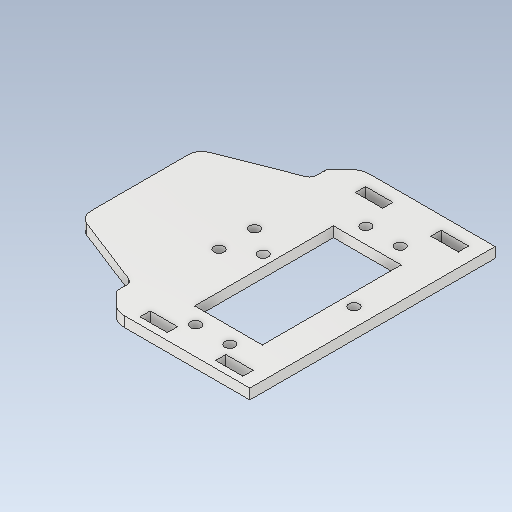
# Autodesk Inventor part: Dock bot2
Saved by Autodesk Inventor 2020.3 (Build 243373000, 373)
## iProperties
Created: 2017-03-28
Part Number: Dock bot2
Material: Acrylic
Document SubType Name: Modeling
Designer: Nanjar
Density: 1.188 g/cm^3
Appearance: Transparent - Clear
Author: Nanjar
Autodesk Inventor part; units mm, degrees
ref_plane "YZ Plane" through (0, 0, 0) normal (1, 0, 0) x (0, 1, 0)
ref_plane "XZ Plane" through (0, 0, 0) normal (0, 1, 0) x (-1, 0, 0)
ref_plane "XY Plane" through (0, 0, 0) normal (0, 0, 1) x (1, 0, 0)
sketch "Sketch1" plane through (0, 0, 0) normal (0, 1, 0) x (-1, 0, 0)
  circle A0 centre (7.7, 5.2) radius 1.5
  circle A1 centre (7.7, -5.2) radius 1.5
  circle A2 centre (0, 0) radius 1.5
  line L0 (37.8003, -0.0084) -> (-30.1744, -0.0084) construction
  line L1 (-27.0022, -36.8848) -> (-27.0022, -0.0084)
  line L2 (12.164, -30.8563) -> (6.1355, -36.8848)
  line L3 (-27.0022, -36.8848) -> (6.1355, -36.8848)
  line L4 (36.1543, -0.0084) -> (36.1543, -17.0084)
  line L5 (36.1543, -17.0084) -> (12.164, -30.8563)
  line L6 (-27.0022, 36.8681) -> (-27.0022, -0.0084)
  line L7 (12.164, 30.8396) -> (6.1355, 36.8681)
  line L8 (-27.0022, 36.8681) -> (6.1355, 36.8681)
  line L9 (36.1543, -0.0084) -> (36.1543, 16.9916)
  line L10 (36.1543, 16.9916) -> (12.164, 30.8396)
  constraints: 22 end point, 4 symmetric about line, 3 centre point, 2 horizontal, 2 point on line, 1 perpendicular, 1 vertical
extrude "Extrusion1" add sketch "Sketch1" along normal blind 3
sketch "Sketch2" plane through (0, 3, 0) normal (0, 1, 0) x (1, 0, 0)
  circle A0 centre (13, 13.115) radius 3.5
  point P0 (0, 0)
  dimension "d2" = 7
  dimension "d3" = 13.115
  dimension "d4" = 13
  constraints: 1 centre point
  measures "d2" diameter of A0
  measures "d3" vertical distance of A0.centre point (0, 0)
  measures "d4" horizontal distance of A0.centre point (0, 0)
extrude "Extrusion2" cut sketch "Sketch2" against normal through all
move faces "Move1" translate (0.9995, 0, 0) faces at (27.0022, 1, -12.3005)
sketch "Sketch5" plane through (0, 0, 0) normal (0, -1, 0) x (1, 0, 0)
  circle A0 centre (18.0046, -22.074) radius 1.5
  circle A1 centre (8.0046, -22.0753) radius 1.5
  circle A2 centre (17.9981, 27.7053) radius 1.5
  circle A3 centre (7.9981, 27.704) radius 1.5
  line L0 (22.8987, 23.1163) -> (22.904, -17.4837)
  line L1 (22.904, -17.4837) -> (3.104, -17.4863)
  line L2 (3.0987, 23.1137) -> (22.8987, 23.1163)
  line L3 (3.104, -17.4863) -> (3.0987, 23.1137)
  point P0 (0, 0)
  constraints: 8 end point, 4 centre point
extrude "Extrusion4" cut sketch "Sketch5" against normal through all
sketch "Sketch6" plane through (0, 3, 0) normal (0, 1, 0) x (1, 0, 0)
  circle A0 centre (0, 0) radius 1.5
  circle A1 centre (26.6, 0) radius 1.5
  dimension "d22" = 3
  dimension "d23" = 26.6
  constraints: 2 centre point
  measures "d22" diameter of A1
  measures "d23" distance of A1.centre A0.centre
move faces "Move2" translate (3.9857, 0, 0) faces at (28.0017, 1, -12.3005)
extrude "Extrusion5" cut sketch "Sketch6" against normal through all
sketch "Sketch7" plane through (0, 3, 0) normal (0, 1, 0) x (1, 0, 0)
  line L0 (27.9874, -33.8681) -> (19.9874, -33.8681)
  line L1 (19.9874, -30.8681) -> (19.9874, -33.8681)
  line L2 (27.9874, -30.8681) -> (27.9874, -33.8681)
  line L3 (19.9874, -30.8681) -> (27.9874, -30.8681)
  line L4 (5.8645, -33.8681) -> (-2.1355, -33.8681)
  line L5 (-2.1355, -30.8681) -> (-2.1355, -33.8681)
  line L6 (-2.1355, -30.8681) -> (5.8645, -30.8681)
  line L7 (5.8645, -30.8681) -> (5.8645, -33.8681)
  line L8 (-2.1355, 32.1319) -> (5.8645, 32.1319)
  line L9 (5.8645, 29.1319) -> (-2.1355, 29.1319)
  line L10 (5.8645, 32.1319) -> (5.8645, 29.1319)
  line L11 (-2.1355, 32.1319) -> (-2.1355, 29.1319)
  line L12 (19.9874, 32.1319) -> (19.9874, 29.1319)
  line L13 (27.9874, 32.1319) -> (27.9874, 29.1319)
  line L14 (27.9874, 29.1319) -> (19.9874, 29.1319)
  line L15 (19.9874, 32.1319) -> (27.9874, 32.1319)
  point P0 (0, 0)
  point P1 (31.9874, -36.8681)
  constraints: 32 end point
extrude "Extrusion6" cut sketch "Sketch7" against normal through all
sketch "Sketch8" plane through (0, 3, 0) normal (0, 1, 0) x (1, 0, 0)
  line L0 (5.8645, -33.8681) -> (-2.1355, -33.8681) projected
  line L1 (-2.1355, -35.8681) -> (-2.1355, -36.8681) construction
  line L2 (-2.1355, 32.1319) -> (5.8645, 32.1319) construction
  line L3 (31.9874, 35.8848) -> (-7.1355, 35.8848)
  line L4 (31.9874, -35.8681) -> (-7.1355, -35.8681)
  line L5 (31.9874, -36.8681) -> (31.9874, -35.8681)
  line L6 (31.9874, 35.8848) -> (31.9874, 36.8848)
  line L7 (-6.1355, 36.8848) -> (-7.1355, 35.8848)
  line L8 (-6.1355, -36.8681) -> (-7.1355, -35.8681)
  line L9 (-6.1355, -36.8681) -> (31.9874, -36.8681)
  line L10 (-6.1355, 36.8848) -> (31.9874, 36.8848)
  point P0 (0, 0)
  dimension "d32" = 2
  constraints: 18 end point, 2 horizontal, 2 vertical
  measures "d32" distance of L0.end L1.start
extrude "Extrusion7" cut sketch "Sketch8" against normal through all
sketch "Sketch9" plane through (0, 3, 0) normal (0, 1, 0) x (1, 0, 0)
  line L0 (-12.164, 30.8563) -> (-12.164, 14.1606) construction
  line L1 (-12.164, 26.3921) -> (-12.164, 30.8563)
  line L2 (-36.1543, 17.0084) -> (-12.164, 30.8563) projected
  line L3 (-36.1543, 17.0084) -> (-12.164, 30.8563)
  line L4 (-36.1543, 17.0084) -> (-12.164, 26.3921)
  line L5 (-41.6853, 0) -> (0, 0) construction
  line L6 (-12.164, -30.8396) -> (-12.164, -14.1438) construction
  line L7 (-12.164, -26.3753) -> (-12.164, -30.8396)
  line L8 (-36.1543, -16.9916) -> (-12.164, -30.8396)
  line L9 (-36.1543, -16.9916) -> (-12.164, -26.3753)
  constraints: 18 end point, 2 collinear, 2 point on line, 1 horizontal, 1 vertical
extrude "Extrusion8" cut sketch "Sketch9" against normal up to next
fillet "Fillet1" radius 6 2 edges at (-7.1355, 1.5, -35.8848) (-7.1355, 1.5, 35.8681)
fillet "Fillet2" radius 2 4 edges at (-12.164, 1.5, -26.3921) (-12.164, 1.5, 26.3753) (-12.164, 1.5, 30.8396) (-12.164, 1.5, -30.8563)
fillet "Fillet3" radius 4 2 edges at (-36.1543, 1.5, 16.9916) (-36.1543, 1.5, -17.0084)
body "Solid1"
